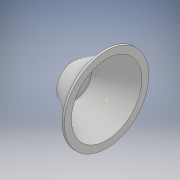
# Autodesk Inventor part: base-biotrap
Saved by Autodesk Inventor 2017 (Build 210142000, 142)
## iProperties
Created: 2018-06-28
Part Number: base-biotrap
Material: Generic
Document SubType Name: Modeling
Designer: 45027374
Density: 1 g/cm^3
Appearance: Default
Author: 45027374
Autodesk Inventor part; units mm, degrees
ref_plane "YZ Plane" through (0, 0, 0) normal (1, 0, 0) x (0, 1, 0)
ref_plane "XZ Plane" through (0, 0, 0) normal (0, 1, 0) x (-1, 0, 0)
ref_plane "XY Plane" through (0, 0, 0) normal (0, 0, 1) x (1, 0, 0)
sketch "Sketch1" plane through (0, 0, 0) normal (0, 1, 0) x (-1, 0, 0)
  point P0 (0, 0)
sketch "Sketch2" plane through (0, 0, 0) normal (0, 1, 0) x (-1, 0, 0)
  line L0 (0, -25) -> (0, -30)
  line L1 (0, -30) -> (1.5, -30)
  line L2 (1.5, -30) -> (1.5, -25.8289)
  line L3 (1.5, -25.8289) -> (23.5, -12)
  line L4 (23.5, -12) -> (23.5, -4.75)
  line L5 (23.5, -4.75) -> (22, -4.75)
  line L6 (22, -4.75) -> (22, -11.1711)
  line L7 (22, -11.1711) -> (0, -25)
  line L8 (28.2, 0) -> (-4.7, 0) projected
  line L9 (0, -36) -> (0, 6) projected
  dimension "d6" = 1.5
  dimension "d7" = 1.5
  dimension "d8" = 4.75
  dimension "d9" = 7.25
  dimension "d10" = 5
  dimension "d11" = 30
  dimension "d12" = 23.5
  dimension "d13" = 1.5
  constraints: 16 end point, 4 perpendicular, 2 parallel, 1 collinear, 1 vertical
  measures "d6" distance of L0.end L1.end
  measures "d7" distance of L4.end L5.end
  measures "d8" distance between parallel lines of L8 L5
  measures "d9" distance of L3.end L4.end
  measures "d10" distance of L0.start L0.end
  measures "d11" distance between parallel lines of L8 L1
  measures "d12" distance between parallel lines of L9 L4
  measures "d13" distance between parallel lines of L7 L3
revolve "Revolution1" add sketch "Sketch2" angle 360 about axis through (-10, 0, 0) along (1, 0, 0)
body "Solid1"
